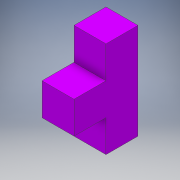
# Autodesk Inventor part: Purple part
Saved by Autodesk Inventor 2017 (Build 210142000, 142)
## iProperties
Created: 2016-11-01
Part Number: Purple part
Material: Generic
Document SubType Name: Modeling
Designer: rbibb
Density: 1 g/cm^3
Appearance: Default
Author: rbibb
Autodesk Inventor part; units mm, degrees
ref_plane "YZ Plane" through (0, 0, 0) normal (1, 0, 0) x (0, 1, 0)
ref_plane "XZ Plane" through (0, 0, 0) normal (0, 1, 0) x (-1, 0, 0)
ref_plane "XY Plane" through (0, 0, 0) normal (0, 0, 1) x (1, 0, 0)
sketch "Sketch1" plane through (0, 0, 0) normal (1, 0, 0) x (0, 1, 0)
  line L0 (12.4105, 20.1975) -> (-44.7395, 20.1975)
  line L1 (-44.7395, 20.1975) -> (-44.7395, 1.1475)
  line L2 (-44.7395, 1.1475) -> (12.4105, 1.1475)
  line L3 (12.4105, 1.1475) -> (12.4105, 20.1975)
  point P0 (0, 0)
  dimension "d0" = 57.15
  dimension "d1" = 19.05
  constraints: 8 end point, 2 parallel, 1 horizontal, 1 perpendicular
  measures "d0" distance of L2.end L1.end
  measures "d1" distance of L1.end L0.end
extrude "Extrusion1" add sketch "Sketch1" along normal blind 19.05
sketch "Sketch2" plane through (0, -44.7395, 20.1975) normal (0, 0, 1) x (1, 0, 0)
  line L0 (0, 57.15) -> (19.05, 57.15) projected
  line L1 (0, 57.15) -> (0, 38.1)
  line L2 (0, 57.15) -> (0, 0) projected
  line L3 (19.05, 57.15) -> (19.05, 0) projected
  line L4 (0, 38.1) -> (19.05, 38.1)
  line L5 (19.05, 38.1) -> (19.05, 19.05)
  line L6 (19.05, 19.05) -> (0, 19.05)
  line L7 (0, 19.05) -> (0, 38.1)
  point P0 (0, 44.7395)
  dimension "d4" = 19.05
  dimension "d5" = 19.05
  constraints: 10 end point, 2 parallel, 2 point on line, 1 horizontal, 1 perpendicular
  measures "d4" distance of L0.start L1.end
  measures "d5" distance of L4.end L5.end
extrude "Extrusion2" add sketch "Sketch2" along normal blind 19.05 contours L4 L3 L6 L2
body "Solid1"
